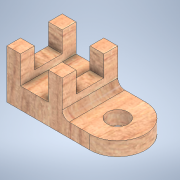
# Autodesk Inventor part: ch3-saddlebracket
Saved by Autodesk Inventor 2020 (Build 240168000, 168)
## iProperties
Created: 2020-02-07
Part Number: ch3-saddlebracket
Material: Wood (Birch)
Document SubType Name: Modeling
Designer: Eric
Mass: 52.6472 g
Surface Area: 202.059 cm^2
Volume: 95.7223 cm^3
Density: 0.55 g/cm^3
Appearance: Birch - Natural Polished
Author: Eric
Autodesk Inventor part; units mm, degrees
ref_plane "YZ Plane" through (0, 0, 0) normal (1, 0, 0) x (0, 1, 0)
ref_plane "XZ Plane" through (0, 0, 0) normal (0, 1, 0) x (-1, 0, 0)
ref_plane "XY Plane" through (0, 0, 0) normal (0, 0, 1) x (1, 0, 0)
sketch "Sketch1" plane through (0, 0, 0) normal (0, 0, 1) x (1, 0, 0)
  line L0 (-38.1, 44.45) -> (-38.1, 0)
  line L1 (-38.1, 0) -> (38.1, 0)
  line L2 (38.1, 0) -> (38.1, 12.7)
  line L3 (38.1, 12.7) -> (19.05, 12.7)
  line L4 (12.7, 19.05) -> (12.7, 44.45)
  line L5 (12.7, 44.45) -> (0, 44.45)
  line L6 (0, 44.45) -> (0, 19.05)
  line L7 (0, 19.05) -> (-25.4, 19.05)
  line L8 (-25.4, 19.05) -> (-25.4, 44.45)
  line L9 (-25.4, 44.45) -> (-38.1, 44.45)
  arc A0 (12.7, 19.05) -> (19.05, 12.7) centre (19.05, 19.05) ccw
  point P0 (12.7, 12.7)
  point P1 (0, 0)
  point P2 (0, 0)
  point P3 (0, 0)
  dimension "d0" = 76.2
  dimension "d1" = 44.45
  dimension "d2" = 12.7
  dimension "d3" = 19.05
  dimension "d4" = 50.8
  dimension "d5" = 12.7
  dimension "d18" = 6.35
  constraints: 20 end point, 9 perpendicular, 3 coincident, 3 point on line, 2 point on circle, 2 tangent, 1 centre point, 1 collinear, 1 midpoint, 1 vertical
  measures "d0" distance of L0.end L1.end
  measures "d1" distance of L0.end L0.start
  measures "d2" distance of L1.end L2.end
  measures "d3" distance between parallel lines of L1 L7
  measures "d4" distance of L4.end L0.start
  measures "d5" distance of L8.end L0.start
  measures "d18" radius of A0
extrude "Extrusion1" add sketch "Sketch1" along normal mid plane 50.8
sketch "Sketch2" plane through (-38.1, 0, 25.4) normal (0, -1, 0) x (1, 0, 0)
  line L0 (76.2, -50.8) -> (76.2, 0) construction
  circle A0 centre (76.2, -25.4) radius 25.4
  point P0 (38.1, -25.4)
  constraints: 1 midpoint, 1 vertical alignment, 2 other
extrude "Extrusion2" add sketch "Sketch2" against normal up to surface (12.7 mm away)
sketch "Sketch5" plane through (12.7, 12.7, 25.4) normal (0, 1, 0) x (1, 0, 0)
  arc A0 (25.4, 0) -> (25.4, 50.8) centre (25.4, 25.4) ccw construction
  point P0 (-12.7, 25.4)
  constraints: 1 coincident
hole "Hole1" at (38.1, 12.7, 0) direction (0, -1, 0) diameter 19.05 end through all
sketch "Sketch6" plane through (12.7, 19.05, 25.4) normal (1, 0, 0) x (0, 0, -1)
  line L0 (50.8, 25.4) -> (0, 25.4) construction
  line L1 (12.7, 25.4) -> (38.1, 25.4)
  line L2 (38.1, 25.4) -> (38.1, 6.35)
  line L3 (38.1, 6.35) -> (12.7, 6.35)
  line L4 (12.7, 6.35) -> (12.7, 25.4)
  point P0 (25.4, -19.05)
  point P1 (25.4, 25.4)
  dimension "d19" = 19.05
  dimension "d20" = 25.4
  constraints: 8 end point, 2 midpoint, 2 parallel, 1 horizontal, 1 perpendicular, 1 point on line
  measures "d19" distance of L3.end L1.start
  measures "d20" distance of L2.end L3.end
extrude "Extrusion3" cut sketch "Sketch6" against normal through all
body "Solid1"
